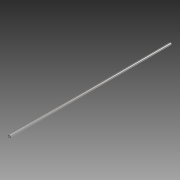
# Autodesk Inventor part: 2315_Shaft_V1
Saved by Autodesk Inventor 2020 (Build 240168000, 168)
## iProperties
Created: 2019-10-13
Part Number: 2315_Shaft_V1
Material: Stainless Steel, Austenitic
Document SubType Name: Modeling
Designer: RFLab
Density: 8 g/cm^3
Appearance: Semi-Polished
Author: RFLab
Autodesk Inventor part; units mm, degrees
ref_plane "YZ Plane" through (0, 0, 0) normal (1, 0, 0) x (0, 1, 0)
ref_plane "XZ Plane" through (0, 0, 0) normal (0, 1, 0) x (-1, 0, 0)
ref_plane "XY Plane" through (0, 0, 0) normal (0, 0, 1) x (1, 0, 0)
sketch "Sketch1" plane through (0, 0, 0) normal (0, 0, 1) x (1, 0, 0)
  circle A0 centre (0, 0) radius 6.35
  dimension "d0" = 12.7
  constraints: 1 centre point, 1 coincident
  measures "d0" diameter of A0
extrude "Extrusion1" add sketch "Sketch1" along normal mid plane 914.4
chamfer "Chamfer1" distance 1 angle 45 2 edges at (-6.35, 0, 457.2) (-6.35, 0, -457.2)
body "Solid1"
